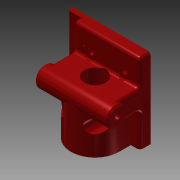
# Autodesk Inventor part: Carraige
Saved by Autodesk Inventor 2015 SP1 (Build 190203100, 203)
## iProperties
Created: 2015-02-03
Part Number: Carraige
Material: Generic
Document SubType Name: Modeling
Designer: Joseph
Density: 1 g/cm^3
Appearance: Red
Author: Joseph
Autodesk Inventor part; units mm, degrees
ref_plane "YZ Plane" through (0, 0, 0) normal (1, 0, 0) x (0, 1, 0)
ref_plane "XZ Plane" through (0, 0, 0) normal (0, 1, 0) x (-1, 0, 0)
sketch "Sketch1" plane through (0, 0, 0) normal (0, 0, 1) x (1, 0, 0)
  line L0 (0, 0) -> (0, 48) projected
  line L1 (0, 0) -> (27, 0) construction
  line L2 (27, 0) -> (27, 48) construction
  line L3 (0, 48) -> (27, 48) construction
  line L4 (20, 24) -> (-20, 24)
  line L5 (-20, 24) -> (-20, -24)
  line L6 (-20, -24) -> (20, -24)
  line L7 (20, -24) -> (20, 24)
  line L8 (20, 24) -> (-20, -24) construction
  line L9 (-20, 24) -> (20, -24) construction
  dimension "d0" = 40
  constraints: 12 end point, 2 midpoint, 2 parallel, 1 coincident, 1 horizontal, 1 perpendicular
  measures "d0" distance of L6.end L5.end
extrude "Extrusion1" add sketch "Sketch1" along normal blind 30
sketch "Sketch5" plane through (-20, -24, 0) normal (-1, 0, 0) x (0, 0, 1)
  line L0 (0, 48) -> (0, 0) projected
  line L1 (0, 0) -> (30, 0) projected
  arc A0 (21.9437, 20.0563) -> (21.9437, 32.0563) centre (21.9437, 26.0563) ccw
  line L2 (0, 48) -> (4.4156, 48)
  line L3 (6.4156, 0) -> (0, 0)
  line L4 (0, 0) -> (0, 48)
  line L5 (21.9437, 32.0563) -> (8.4156, 32.0563)
  line L6 (8.4156, 20.0563) -> (21.9437, 20.0563)
  line L7 (6.4156, 46) -> (6.4156, 34.0563)
  line L8 (6.4156, 18.0563) -> (6.4156, 0)
  arc A1 (6.4156, 34.0563) -> (8.4156, 32.0563) centre (8.4156, 34.0563) ccw
  arc A2 (8.4156, 20.0563) -> (6.4156, 18.0563) centre (8.4156, 18.0563) ccw
  arc A3 (6.4156, 46) -> (4.4156, 48) centre (4.4156, 46) ccw
  dimension "d19" = 2
  dimension "d20" = 2
  dimension "d37" = 6
  constraints: 14 end point, 8 point on circle, 6 tangent, 4 centre point, 4 parallel, 2 horizontal, 2 perpendicular, 1 equal radius, 1 point on line
  measures "d19" radius of A1
  measures "d20" radius of A3
  measures "d37" radius of A0
extrude "Extrusion5" cut sketch "Sketch5" against normal through all keep common part
sketch "Sketch6" plane through (-20, -24, 0) normal (0, -1, 0) x (1, 0, 0)
  line L0 (12.4815, -9.7926) -> (5.5063, 0) construction
  line L1 (47, 0) -> (47, -10) construction
  line L2 (5.5063, 0) -> (34.4937, 0)
  line L3 (34.4937, 0) -> (34.4937, 13.45)
  line L4 (5.5063, 13.45) -> (5.5063, 0)
  arc A0 (34.4937, 13.45) -> (5.5063, 13.45) centre (20, 13.45) ccw
  circle A1 centre (20, 13.45) radius 6.5
  line L5 (20, 13.45) -> (20, 0) construction
  line L6 (0, 6.4156) -> (40, 6.4156)
  line L7 (0, 0) -> (40, 0)
  line L8 (0, 0) -> (40, 0) projected
  line L9 (0, 27.9437) -> (40, 27.9437) construction
  point P0 (20.781, 27.9226)
  dimension "d23" = 13
  dimension "d24" = 13.45
  constraints: 14 end point, 3 midpoint, 3 point on circle, 2 centre point, 2 tangent, 1 coincident, 1 horizontal, 1 parallel, 1 perpendicular, 1 vertical
  measures "d23" diameter of A1
  measures "d24" distance of L5.start L5.end
extrude "Extrusion6" add sketch "Sketch6" against normal up to next
sketch "Sketch2" plane through (-20, -24, 0) normal (-1, 0, 0) x (0, 0, 1)
  line L0 (0, 48) -> (0, 0) projected
  circle A0 centre (21.9437, 26.0563) radius 1.5
  line L1 (-3.5, 32.7705) -> (0, 32.7705) construction
  line L2 (-3.5, 15.2295) -> (0, 15.2295) construction
  line L3 (0, 32.7705) -> (0, 15.2295) construction
  line L4 (0, 52.771) -> (2, 52.771) construction
  line L5 (2, 52.771) -> (2, -5.2729) construction
  line L6 (2, -5.2729) -> (0, -5.2729) construction
  line L7 (0, -5.2729) -> (0, 52.771) construction
  line L8 (2, 49.5092) -> (13, 49.5092) construction
  line L9 (13, 49.5092) -> (13, -2.3456) construction
  line L10 (13, -2.3456) -> (2, -2.3456) construction
  line L11 (2, -2.3456) -> (2, 49.5092) construction
  line L12 (21.9437, 20.0563) -> (8.4156, 20.0563)
  arc A1 (21.9437, 20.0563) -> (21.9437, 32.0563) centre (21.9437, 26.0563) ccw projected
  dimension "d3" = 3
  dimension "d14" = 2
  dimension "d15" = 11
  constraints: 24 end point, 4 horizontal, 4 parallel, 2 perpendicular, 1 centre point, 1 coincident, 1 collinear, 1 point on line, 4 other
  measures "d3" diameter of A0
  measures "d14" distance of L5.end L6.end
  measures "d15" distance of L9.end L10.end
extrude "Extrusion2" cut sketch "Sketch2" against normal through all
sketch "Sketch10" plane through (0, 0, 0) normal (1, 0, 0) x (0, 1, 0)
  circle A0 centre (2.0563, 21.9437) radius 1.5 projected
  arc A1 (8.0563, 21.9437) -> (-3.9437, 21.9437) centre (2.0563, 21.9437) ccw construction
  circle A2 centre (2.0563, 21.9437) radius 6
  point P0 (0, 0)
  constraints: 1 centre point, 1 coincident, 1 concentric
extrude "Extrusion8" add sketch "Sketch10" along normal mid plane 44
sketch "Sketch3" plane through (-20, -24, 0) normal (-1, 0, 0) x (0, 0, 1)
  line L0 (0, 0) -> (30, 0) projected
  line L1 (0, 48) -> (1, 48)
  line L2 (2, 47) -> (2, 1)
  line L3 (1, 0) -> (0, 0)
  line L4 (0, 0) -> (0, 48)
  line L5 (1, 48) -> (2, 47)
  line L6 (2, 1) -> (1, 0)
  point P0 (2, 0)
  point P1 (2, 48)
  dimension "d7" = 2
  dimension "d8" = 1
  dimension "d9" = 1
  dimension "d10" = 1
  dimension "d11" = 1
  constraints: 12 end point, 5 point on line, 2 parallel, 1 horizontal, 1 perpendicular
  measures "d7" distance of point (2, 0) L3.end
  measures "d8" distance of L1.end point (2, 48)
  measures "d9" distance of L2.start point (2, 48)
  measures "d10" distance of L2.end point (2, 0)
  measures "d11" distance of L3.start point (2, 0)
extrude "Extrusion3" add sketch "Sketch3" along normal blind 7
sketch "Sketch7" plane through (20, -24, 0) normal (0, -1, 0) x (1, 0, 0)
  circle A0 centre (-20, 13.45) radius 6.5 projected
  arc A1 (-5.5063, 13.45) -> (-34.4937, 13.45) centre (-20, 13.45) ccw projected
  circle A2 centre (-20, 13.45) radius 6.5
  point P0 (-20, 0)
  constraints: 1 centre point, 1 coincident, 1 concentric
extrude "Extrusion7" cut sketch "Sketch7" against normal through all
ref_plane "Work Plane1" through (-20, 2.0563, 27.9437) normal (0, 0, -1) x (-1, 0, 0)
sketch "Sketch8" plane through (-20, 2.0563, 27.9437) normal (0, 0, -1) x (-1, 0, 0)
  circle A0 centre (-10, 10) radius 1.2295 construction
  circle A1 centre (-30, 10) radius 1.2295 construction
  circle A2 centre (-30, -10) radius 1.2295 construction
  circle A3 centre (-10, -10) radius 1.2295 construction
  line L0 (-10, 10) -> (-30, 10) construction
  line L1 (-30, 10) -> (-30, -10) construction
  line L2 (-30, -10) -> (-10, -10) construction
  line L3 (-10, -10) -> (-10, 10) construction
  circle A4 centre (-20, 0) radius 10 construction
  point P0 (-20, 0)
  dimension "d49" = 20
  constraints: 8 end point, 7 coincident, 5 centre point, 3 tangent, 2 parallel, 2 perpendicular, 1 horizontal
  measures "d49" distance of L2.end L0.start
hole "Hole1" at (-10, 12.0563, 27.9437) at (10, 12.0563, 27.9437) at (10, -7.9437, 27.9437) at (-10, -7.9437, 27.9437) direction (0, 0, -1) diameter 3.4 end through all counterbore diameter 8 counterbore depth 22 clearance for "Socket Head Cap Screw" size "M3" standard "Ansi Metric M Profile"
sketch "Sketch9" plane through (-27, -24, 0) normal (0, -1, 0) x (1, 0, 0)
  arc A0 (41.4937, 13.45) -> (12.5063, 13.45) centre (27, 13.45) ccw projected
  circle A1 centre (21.1466, 6.0618) radius 1.2295 construction
  circle A2 centre (23.0749, 21.9452) radius 1.2295 construction
  circle A3 centre (35.8662, 12.3335) radius 1.2295 construction
  circle A4 centre (27, 13.45) radius 9.3581 construction
  line L0 (27, 22.8081) -> (18.8956, 8.7709) construction
  line L1 (35.1044, 8.7709) -> (18.8956, 8.7709) construction
  line L2 (35.1044, 8.7709) -> (27, 22.8081) construction
  point P0 (27, 0)
  constraints: 6 end point, 4 coincident, 4 point on circle, 2 equal length, 1 centre point, 1 horizontal
hole "Hole2" at (0, -24, 22.8081) at (-8.1044, -24, 8.7709) at (8.1044, -24, 8.7709) direction (0, 1, 0) diameter 2.459 depth 8.8 tip angle 118 thread size "M3x0.5" class "6H" standard "ANSI Metric M Profile"
chamfer "Chamfer2" distance 1 angle 45 2 edges at (22, -3.9437, 21.9437) (-22, -3.9437, 21.9437)
fillet "Fillet3" radius 2 16 edges at (20, 8.6421, 7.0014) (20, 16.0282, 6.4156) (20, 23.4142, 5.8298) (20, 24, 2.2078) (20, 8.0563, 15.1796) (20, -4.5295, 7.0014) (20, -3.9437, 15.1796) (20, -14.9718, 6.4156) (-20, 8.6421, 7.0014) (-20, 16.0282, 6.4156) (-20, 23.4142, 5.8298) (-20, 24, 2.7078) (-20, 8.0563, 15.1796) (-20, -4.5295, 7.0014) (-20, -14.9718, 6.4156) (-20, -3.9437, 15.1796)
equation "\"d9\" = d8"
equation "\"d10\" = d8"
equation "\"d11\" = d10"
body "Solid1"
